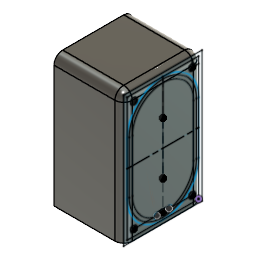
Speaker Mount (Autodesk Fusion 360 design; units mm, degrees)
Autodesk Fusion 360 part; units mm, degrees
sketch "Sketch1" plane through (0, 0, 0) normal (1, 0, 0) x (0, 1, 0)
  line L0 (0, 0) -> (-41, 0)
  line L1 (-41, 0) -> (-41, 71)
  line L2 (-41, 71) -> (0, 71)
  line L3 (0, 71) -> (0, 0)
  line L4 (-20.5, 71) -> (-20.5, 50.5)
  line L5 (-41, 35.5) -> (0, 35.5)
  line L6 (-38, 50.5) -> (-38, 20.5)
  arc A0 (-38, 20.5) -> (-3, 20.5) centre (-20.5, 20.5) ccw
  line L7 (-3, 20.5) -> (-3, 50.5)
  arc A1 (-3, 50.5) -> (-38, 50.5) centre (-20.5, 50.5) ccw
  line L8 (-20.5, 50.5) -> (-20.5, 20.5) construction
  line L9 (-39.7873, 50.5) -> (-39.7873, 20.5)
  arc A2 (-39.7873, 20.5) -> (-1.2127, 20.5) centre (-20.5, 20.5) ccw
  line L10 (-1.2127, 20.5) -> (-1.2127, 50.5)
  arc A3 (-1.2127, 50.5) -> (-39.7873, 50.5) centre (-20.5, 50.5) ccw
  line L11 (-20.5, 50.5) -> (-20.5, 20.5) construction
  line L12 (-3.75, 71) -> (-3.75, 67.25)
  line L13 (0, 67.25) -> (-3.75, 67.25)
  circle A4 centre (-3.75, 67.25) radius 1.75
  circle A5 centre (-37.25, 67.25) radius 1.75
  circle A6 centre (-37.25, 3.75) radius 1.75
  circle A7 centre (-3.75, 3.75) radius 1.75
  line L14 (-20.5, 71) -> (-20.5, 0) construction
  line L15 (2, -2) -> (-43, -2)
  line L16 (-43, -2) -> (-43, 73)
  line L17 (-43, 73) -> (2, 73)
  line L18 (2, 73) -> (2, -2)
  line L19 (-41, 50.5) -> (-41, 20.5)
  arc A8 (-41, 20.5) -> (0, 20.5) centre (-20.5, 20.5) ccw
  line L20 (0, 20.5) -> (0, 50.5)
  arc A9 (0, 50.5) -> (-41, 50.5) centre (-20.5, 50.5) ccw
  line L21 (-20.5, 50.5) -> (-20.5, 20.5) construction
  line L22 (-37.25, 3.75) -> (-3.75, 3.75)
  line L23 (-24, 2.25) -> (-17, 2.25)
  arc A10 (-17, 2.25) -> (-17, 5.25) centre (-17, 3.75) ccw
  line L24 (-17, 5.25) -> (-24, 5.25)
  arc A11 (-24, 5.25) -> (-24, 2.25) centre (-24, 3.75) ccw
  line L25 (-24, 3.75) -> (-17, 3.75) construction
  point P0 (-20.5, 3.75)
  dimension "d1" = 41
  dimension "d2" = 71
  dimension "d3" = 20.5
  dimension "d4" = 35
  dimension "d5" = 3.75
  dimension "d6" = 3.75
  dimension "d7" = 3.5
  dimension "d8" = 1.7873
  dimension "d9" = 30
  dimension "d10" = -2
  dimension "d27" = 3
  constraint horizontal L0
  constraint vertical L1
  constraint horizontal L2
  constraint vertical L3
  constraint coincident L0.start L3.end
  constraint midpoint L2 L4.start
  constraint perpendicular L2 L4
  constraint midpoint L1 L5.start
  constraint midpoint L3 L5.end
  constraint tangent L6 A0
  constraint tangent A0 L7
  constraint parallel L6 L7
  constraint tangent L7 A1
  constraint tangent L6 A1
  constraint perpendicular L5 L8
  constraint tangent L9 A2
  constraint tangent A2 L10
  constraint parallel L9 L10
  constraint tangent L10 A3
  constraint tangent L9 A3
  constraint coincident A0.centre L8.end
  constraint perpendicular L5 L11
  constraint coincident L2 L12.start
  constraint coincident L3 L13.start
  constraint coincident L12 L13.end
  constraint coincident L12.end L13
  constraint coincident L12.end L13.end
  constraint symmetric L8 A4 A5
  constraint symmetric L5 A4 A7
  constraint symmetric L5 A5 A6
  constraint midpoint L0 L14.end
  constraint concentric A1 A3
  constraint coincident L4.end A1.centre
  constraint perpendicular L12 L13
  constraint horizontal L13
  constraint tangent L19 A8
  constraint tangent A8 L20
  constraint parallel L19 L20
  constraint tangent L20 A9
  constraint tangent L19 A9
  constraint parallel L11 L21
  constraint coincident A6.centre L22.start
  constraint coincident A7.centre L22.end
  constraint tangent L23 A10
  constraint tangent A10 L24
  constraint parallel L23 L24
  constraint tangent L24 A11
  constraint tangent L23 A11
  constraint coincident L22 A10.centre
  constraint perpendicular L14 L25
  constraint midpoint L22 P0
  constraint midpoint L25 P0
  measures "d1" distance of L0.start L0.end
  measures "d2" distance of L0.start L2.end
  measures "d3" distance of L4.start L4.end
  measures "d4" diameter of A0
  measures "d5" distance of L12.start L12.end
  measures "d6" distance of L13.start L12.end
  measures "d7" diameter of A4
  measures "d8" distance of A0 A2
  measures "d9" vertical distance of L4.end A0.centre
  measures "d27" diameter of A10
extrude "Extrude1" add sketch "Sketch1" against normal blind 40 contours L0 L3 A8 | L0 L1 A8 | L2 L3 L12 L13 A4 A9 | L2 L3 L12 L13 A4 | L1 L2 A9 | L15 L16 L17 L18
extrude "Extrude2" add sketch "Sketch1" against normal blind 3 contours A2 A8 L22 | L3 L5 A2 L10 A8 L20 L22 | L1 L5 L9 A2 L19 A8 L22 | L3 L4 L5 L10 A3 L20 A9 | A0 A2 L22 L23 A10 A11 | L5 L6 A0 L9 A2 L22 | L5 A0 L7 A2 L10 L22 | L4 L5 L7 A1 L10 A3 | L1 L4 L5 L9 A3 L19 A9 | A0 L22 A11 | L5 L6 A0 L7 L22 A10 L24 A11 | A0 L22 A10 | L5 L6 L7 A1 | L4 L5 L6 A1 L9 A3 | A0 L22 A10 A11 | A0 L23 A10 A11 | L22 A10 L24 A11 | L12 L13 A4 | L12 L13 A4 | A5 | A6 | A7
fillet "Fillet2" radius 15.5 4 edges at (-3, -20.5, 0) (-3, 0, 35.5) (-3, -20.5, 71) (-3, -41, 35.5)
fillet "Fillet1" radius 5 2 edges at (-20, 2, 73) (-20, -43, 73)
fillet "Fillet3" radius 5 5 edges at (0, -43, 33) (0, -41.5355, 71.5355) (0, -20.5, 73) (0, 0.5355, 71.5355) (0, 2, 33)
sketch "Sketch2" plane through (-40, 0, 0) normal (-1, 0, 0) x (0, -1, 0)
  arc A0 (43, 68) -> (38, 73) centre (38, 68) ccw
  line L0 (38, 73) -> (3, 73)
  arc A1 (3, 73) -> (-2, 68) centre (3, 68) ccw
  line L1 (-2, 68) -> (-2, -2)
  line L2 (-2, -2) -> (43, -2)
  line L3 (43, -2) -> (43, 68)
  arc A2 (41, 50.5) -> (0, 50.5) centre (20.5, 50.5) ccw
  line L4 (41, 50.5) -> (41, 20.5)
  arc A3 (0, 20.5) -> (41, 20.5) centre (20.5, 20.5) ccw
  line L5 (0, 20.5) -> (0, 50.5)
  circle A4 centre (3.75, 3.75) radius 1.75
  circle A5 centre (37.25, 3.75) radius 1.75
  circle A6 centre (37.25, 67.25) radius 1.75
  circle A7 centre (3.75, 67.25) radius 1.75
  circle A8 centre (3.75, 67.25) radius 1.35
  circle A9 centre (3.75, 3.75) radius 1.35
  circle A10 centre (37.25, 3.75) radius 1.35 construction
  circle A11 centre (37.25, 67.25) radius 1.35 construction
  circle A12 centre (37.25, 67.25) radius 1.75
  circle A13 centre (37.25, 3.75) radius 1.75
  circle A14 centre (3.75, 3.75) radius 1.75
  circle A15 centre (3.75, 67.25) radius 1.75
  circle A16 centre (37.25, 3.75) radius 1.35
  circle A17 centre (37.25, 67.25) radius 1.35
  dimension "d21" = 2.7
  dimension "d22" = 2.7
  dimension "d23" = 2.7
  dimension "d24" = 2.7
  constraint concentric A7 A8
  constraint concentric A4 A9
  constraint concentric A5 A10
  constraint concentric A6 A11
  constraint concentric A11 A12
  constraint concentric A10 A13
  constraint concentric A9 A14
  constraint concentric A8 A15
  constraint concentric A10 A16
  constraint concentric A11 A17
  measures "d21" diameter of A8
  measures "d22" diameter of A9
  measures "d23" diameter of A10
  measures "d24" diameter of A11
extrude "Extrude3" add sketch "Sketch2" against normal blind 35 contours A4 A14 | A5 A13 | A6 A12 | A7 A15
extrude "Extrude4" cut sketch "Sketch1" against normal blind 39 contours A0 L22 A10 A11 | A0 L23 A10 A11 | L22 A10 L24 A11
equation "d3 = ( 41 / 2 ) * 1 mm"
equation "d5 = 2 mm + ( 3.5 / 2 ) * 1 mm"
equation "d6 = 2 mm + ( ( 3.5 / 2 ) * 1 mm )"
